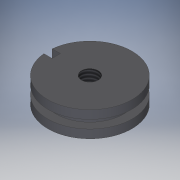
# Autodesk Inventor part: Polia
Saved by Autodesk Inventor 2018 (Build 220112000, 112)
## iProperties
Created: 2017-05-31
Part Number: Polia
Material: Genérico
Document SubType Name: Modeling
Designer: Vitor
Density: 1 g/cm^3
Appearance: Padrão
Author: Vitor
Autodesk Inventor part; units mm, degrees
ref_plane "YZ Plane" through (0, 0, 0) normal (1, 0, 0) x (0, 1, 0)
ref_plane "XZ Plane" through (0, 0, 0) normal (0, 1, 0) x (-1, 0, 0)
ref_plane "XY Plane" through (0, 0, 0) normal (0, 0, 1) x (1, 0, 0)
sketch "Esboço1" plane through (0, 0, 0) normal (0, 0, 1) x (1, 0, 0)
  circle A0 centre (0, 0) radius 5
  dimension "d0" = 10
  constraints: 1 centre point, 1 coincident
  measures "d0" diameter of A0
extrude "Extrusão1" add sketch "Esboço1" along normal blind 1
sketch "Esboço2" plane through (0, 0, 1) normal (0, 0, 1) x (1, 0, 0)
  circle A0 centre (0, 0) radius 4
  dimension "d3" = 8
  constraints: 1 centre point, 1 coincident
  measures "d3" diameter of A0
extrude "Extrusão2" add sketch "Esboço2" along normal blind 1
sketch "Esboço3" plane through (0, 0, 2) normal (0, 0, 1) x (1, 0, 0)
  circle A0 centre (0, 0) radius 5
  dimension "d6" = 10
  constraints: 1 centre point, 1 coincident
  measures "d6" diameter of A0
extrude "Extrusão3" add sketch "Esboço3" along normal blind 1
sketch "Esboço4" plane through (0, 0, 3) normal (0, 0, 1) x (1, 0, 0)
  circle A0 centre (0, 0) radius 4 projected
  circle A1 centre (0, 0) radius 1
  dimension "d9" = 2
  constraints: 1 centre point, 1 coincident
  measures "d9" diameter of A1
extrude "Extrusão4" cut sketch "Esboço4" against normal blind 4 contours A1
thread "Rosca1" size "M2x0.4" class "6H" standard "ANSI Metric M Profile" full length
sketch "Esboço5" plane through (0, 0, 3) normal (0, 0, 1) x (1, 0, 0)
  circle A0 centre (0, 0) radius 5 projected
  line L0 (-4, 0) -> (-4, -0.5)
  circle A1 centre (0, 0) radius 4 projected
  line L1 (-4, 0) -> (-3.5, 0) construction
  line L2 (-4, -0.5) -> (-5, -0.5)
  line L3 (-5, -0.5) -> (-5, 0.5)
  line L4 (-5, -0.5) -> (-4, -0.5) construction
  line L5 (-5, 0.5) -> (-4, 0.5)
  line L6 (-4, 0.5) -> (-4, 0)
  line L7 (-4, -0.5) -> (-5, -0.5)
  dimension "d15" = 0.5
  dimension "d16" = 90
  dimension "d17" = 1
  dimension "d18" = 90
  constraints: 16 end point, 6 perpendicular, 3 vertical, 2 horizontal, 1 collinear, 1 horizontal alignment
  measures "d15" distance of L0.start L0.end
  measures "d16" angle of L0 L1
  measures "d17" distance of L2.end L3.end
  measures "d18" angle of L4 L3
extrude "Extrusão5" cut sketch "Esboço5" against normal blind 10 contours L5 L6 L0 L2 A0 | A0 L3 L5 | L2 L3 A0 picked at (-4.3296, -0.2779)
